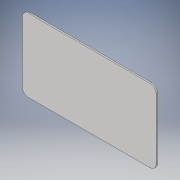
# Autodesk Inventor part: campbellPlacard
Saved by Autodesk Inventor 2017 (Build 210142000, 142)
## iProperties
Created: 2017-04-11
Part Number: campbellPlacard
Material: Generic
Document SubType Name: Sheet Metal
Designer: admin
Density: 1 g/cm^3
Sheet Metal Rule: Default
Appearance: Default
Author: admin
Autodesk Inventor part; units mm, degrees
ref_plane "YZ Plane" through (0, 0, 0) normal (1, 0, 0) x (0, 1, 0)
ref_plane "XZ Plane" through (0, 0, 0) normal (0, 1, 0) x (-1, 0, 0)
ref_plane "XY Plane" through (0, 0, 0) normal (0, 0, 1) x (1, 0, 0)
sketch "Sketch1" plane through (0, 0, 0) normal (0, 0, 1) x (1, 0, 0)
  line L0 (12.7, 0) -> (266.7, 0)
  line L1 (279.4, 12.7) -> (279.4, 139.7)
  line L2 (266.7, 152.4) -> (12.7, 152.4)
  line L3 (0, 139.7) -> (0, 12.7)
  arc A0 (12.7, 152.4) -> (0, 139.7) centre (12.7, 139.7) ccw
  arc A1 (279.4, 139.7) -> (266.7, 152.4) centre (266.7, 139.7) ccw
  arc A2 (266.7, 0) -> (279.4, 12.7) centre (266.7, 12.7) ccw
  arc A3 (0, 12.7) -> (12.7, 0) centre (12.7, 12.7) ccw
  point P0 (0, 0)
  point P1 (279.4, 152.4)
  point P2 (0, 152.4)
  dimension "d0" = 0
  dimension "d1" = 0
  dimension "d2" = 279.4
  dimension "d3" = 152.4
  dimension "d4" = 279.4
  dimension "d5" = 12.7
  measures "d0" distance from line of point (0, 0) L3
  measures "d1" distance from line of L0 point (0, 0)
  measures "d2" distance of point (279.4, 152.4) point (0, 152.4)
  measures "d3" distance between parallel lines of L2 L0
  measures "d4" distance between parallel lines of L3 L1
  measures "d5" radius of A0
extrude "Plate1" add sketch "Sketch1" along normal blind 3.175
equation "\"BendRadius\" = Thickness"
equation "\"BendReliefWidth\" = Thickness"
equation "\"BendReliefDepth\" = 0.5 * Thickness"
equation "\"CornerReliefSize\" = 4 * Thickness"
equation "\"MinimumRemnant\" = 2 * Thickness"
equation "\"TransitionRadius\" = BendRadius"
equation "\"JacobiRadiusSize\" = Thickness"
equation "\"GapSize\" = Thickness"
equation "\"d6\" = BendRadius"
equation "\"Thickness\" = 3.175"
body "Solid1"
